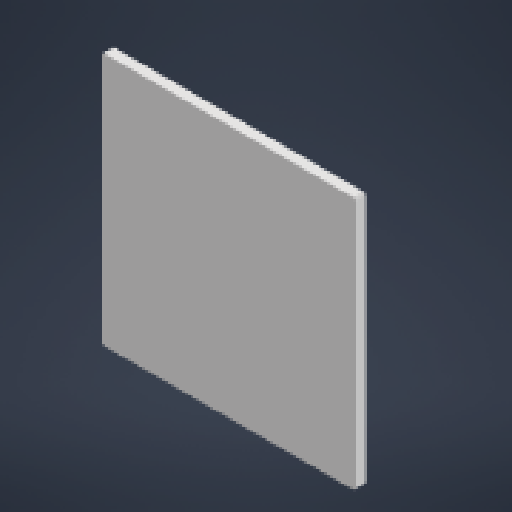
# Autodesk Inventor part: Base stand
Saved by Autodesk Inventor 2026.1 (Build 301233020, 233B)
## iProperties
Created: 2025-12-03
Part Number: Base stand
Material: Generic
Document SubType Name: Modeling
Designer: Mikke
Density: 1 g/cm^3
Appearance: Default
Author: Mikke
Autodesk Inventor part; units mm, degrees
ref_plane "YZ Plane" through (0, 0, 0) normal (1, 0, 0) x (0, 1, 0)
ref_plane "XZ Plane" through (0, 0, 0) normal (0, 1, 0) x (-1, 0, 0)
ref_plane "XY Plane" through (0, 0, 0) normal (0, 0, 1) x (1, 0, 0)
sketch "Sketch1" plane through (0, 0, 0) normal (0, 0, 1) x (1, 0, 0)
  line L0 (20.5, -20.5) -> (20.5, -28.5) projected
  line L1 (28.5, -20.5) -> (20.5, -20.5) projected
  line L2 (28.5, 20.5) -> (28.5, -20.5) projected
  line L3 (20.5, 20.5) -> (28.5, 20.5) projected
  line L4 (20.5, 28.5) -> (20.5, 20.5) projected
  line L5 (-20.5, 28.5) -> (20.5, 28.5) projected
  line L6 (-20.5, 20.5) -> (-20.5, 28.5) projected
  line L7 (-28.5, 20.5) -> (-20.5, 20.5) projected
  line L8 (-28.5, -20.5) -> (-28.5, 20.5) projected
  line L9 (-20.5, -20.5) -> (-28.5, -20.5) projected
  line L10 (-20.5, -28.5) -> (-20.5, -20.5) projected
  line L11 (20.5, -28.5) -> (-20.5, -28.5) projected
  line L12 (-100, -100) -> (100, -100)
  line L13 (100, -100) -> (100, 100)
  line L14 (100, 100) -> (-100, 100)
  line L15 (-100, 100) -> (-100, -100)
  line L16 (-100, -100) -> (100, 100) construction
  line L17 (100, -100) -> (-100, 100) construction
  point P0 (0, 0)
  dimension "d0" = 200
  dimension "d1" = 200
  constraints: 12 end point, 2 midpoint, 2 parallel, 1 horizontal, 1 perpendicular
  measures "d0" distance of L14.end L13.end
  measures "d1" distance of L13.end L12.end
extrude "Extrusion1" add sketch "Sketch1" along normal blind 8 contours L0 L11 L10 L9 L8 L7 L6 L5 L4 L3 L2 L1 | L15 L14 L13 L12
sketch "Sketch2" plane through (0, 0, 0) normal (0, 0, -1) x (-1, 0, 0)
  line L0 (28.5, -20.5) -> (28.5, 20.5) projected
  line L1 (28.5, 20.5) -> (20.5, 20.5) projected
  line L2 (20.5, 20.5) -> (20.5, 28.5) projected
  line L3 (20.5, 28.5) -> (-20.5, 28.5) projected
  line L4 (-20.5, 28.5) -> (-20.5, 20.5) projected
  line L5 (-20.5, 20.5) -> (-28.5, 20.5) projected
  line L6 (-28.5, 20.5) -> (-28.5, -20.5) projected
  line L7 (-28.5, -20.5) -> (-20.5, -20.5) construction
  line L8 (-20.5, -20.5) -> (-20.5, -28.5) construction
  line L9 (-28.5, -20.5) -> (-20.5, -20.5) construction
  line L10 (-28.5, -20.5) -> (-20.5, -20.5) construction
  line L11 (-20.5, -28.5) -> (20.5, -28.5) construction
  line L12 (20.5, -20.5) -> (28.5, -20.5) projected
  line L13 (20.5, -28.5) -> (20.5, -20.5) projected
  line L14 (-35, 35) -> (35, 35)
  line L15 (35, 35) -> (35, -35)
  line L16 (35, -35) -> (-35, -35)
  line L17 (-35, -35) -> (-35, 35)
  line L18 (-35, 35) -> (35, -35) construction
  line L19 (35, 35) -> (-35, -35) construction
  line L20 (-21, -29) -> (-21, -21)
  line L21 (-21, -21) -> (-29, -21)
  line L22 (-29, -21) -> (-29, 21)
  line L23 (-29, 21) -> (-21, 21)
  line L24 (-21, 21) -> (-21, 29)
  line L25 (-21, 29) -> (21, 29)
  line L26 (21, 29) -> (21, 21)
  line L27 (21, 21) -> (29, 21)
  line L28 (29, 21) -> (29, -21)
  line L29 (29, -21) -> (21, -21)
  line L30 (21, -21) -> (21, -29)
  line L31 (21, -29) -> (-21, -29)
  point P0 (0, 0)
  dimension "d4" = 70
  dimension "d5" = 70
  dimension "d6" = 0.5
  constraints: 36 end point, 2 midpoint, 2 parallel, 1 horizontal, 1 perpendicular, 11 other
  measures "d4" distance of L15.end L16.end
  measures "d5" distance of L14.end L15.end
  measures "d6" distance between parallel lines of L8 L20
extrude "Extrusion2" add sketch "Sketch2" along normal blind 35
sketch "Sketch3" plane through (0, 0, -35) normal (0, 0, -1) x (-1, 0, 0)
  line L0 (-35, -35) -> (35, -35) projected
  line L1 (35, -35) -> (35, 35) projected
  line L2 (35, 35) -> (-35, 35) projected
  line L3 (-35, 35) -> (-35, -35) projected
  line L4 (-21, -29) -> (-21, -21) projected
  line L5 (-21, -21) -> (-29, -21) projected
  line L6 (-29, -21) -> (-29, 21) projected
  line L7 (-29, 21) -> (-21, 21) projected
  line L8 (-21, 21) -> (-21, 29) projected
  line L9 (-21, 29) -> (21, 29) projected
  line L10 (21, 29) -> (21, 21) projected
  line L11 (21, 21) -> (29, 21) projected
  line L12 (29, 21) -> (29, -21) projected
  line L13 (29, -21) -> (21, -21) projected
  line L14 (21, -21) -> (21, -29) projected
  line L15 (21, -29) -> (-21, -29) projected
  line L16 (-29, 0) -> (-29, 10)
  line L17 (-29, -21) -> (-29, 21) projected
  line L18 (-29, 10) -> (-29, -10)
  line L19 (-29, 10) -> (-35, 10)
  line L20 (-35, 10) -> (-35, -10)
  line L21 (-35, -10) -> (-29, -10)
  line L22 (-29, -10) -> (-29, 10)
  point P0 (0, 0)
  dimension "d9" = 10
  dimension "d10" = 20
  constraints: 12 end point, 3 point on line, 2 parallel, 1 horizontal, 1 midpoint, 1 perpendicular
  measures "d9" distance of L16.start L16.end
  measures "d10" distance of L16.end L18.end
extrude "Extrusion3" cut sketch "Sketch3" against normal blind 35 contours L3 L19 L6 L21
chamfer "Chamfer1" distance 19.4625 angle 45 5 edges at (35, 22.5, 0) (35, -22.5, 0) (0, -35, 0) (-35, 0, 0) (0, 35, 0)
sketch "Sketch4" plane through (0, 0, -35) normal (0, 0, -1) x (-1, 0, 0)
  circle A0 centre (24.5, 24.5) radius 2.5 projected
  circle A1 centre (24.5, -24.5) radius 2.5 projected
  circle A2 centre (-24.5, -24.5) radius 2.5 projected
  circle A3 centre (-24.5, 24.5) radius 2.5 projected
  circle A4 centre (24.5, 24.5) radius 3
  circle A5 centre (-24.5, 24.5) radius 3
  circle A6 centre (-24.5, -24.5) radius 3
  circle A7 centre (24.5, -24.5) radius 3
  point P0 (0, 0)
  dimension "d16" = 6
  dimension "d17" = 6
  dimension "d18" = 6
  dimension "d19" = 6
  constraints: 4 centre point, 4 coincident
  measures "d16" diameter of A4
  measures "d17" diameter of A5
  measures "d18" diameter of A6
  measures "d19" diameter of A7
extrude "Extrusion4" cut sketch "Sketch4" against normal blind 10 contours A0 | A1 | A2 | A3 | A4 | A5 | A6 | A7
fillet "Fillet1" radius 2 4 edges at (100, 100, 4) (100, -100, 4) (-100, -100, 4) (-100, 100, 4)
body "Solid1"
